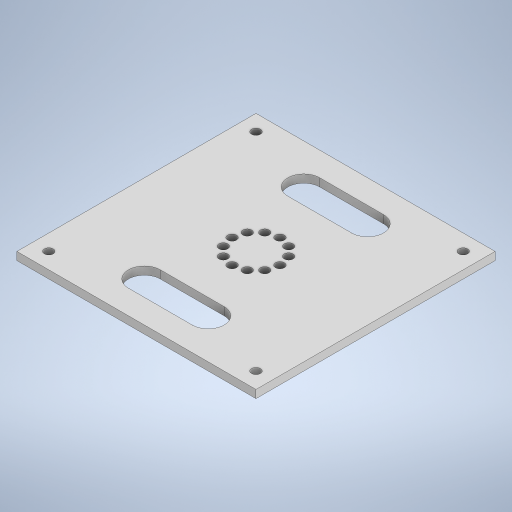
# Autodesk Inventor part: LowerBase
Saved by Autodesk Inventor 2023 (Build 270158000, 158)
## iProperties
Created: 2023-12-19
Part Number: LowerBase
Material: Generic
Document SubType Name: Modeling
Designer: Mustapha
Density: 1 g/cm^3
Appearance: Default
Author: Mustapha
Autodesk Inventor part; units mm, degrees
ref_plane "YZ Plane" through (0, 0, 0) normal (1, 0, 0) x (0, 1, 0)
ref_plane "XZ Plane" through (0, 0, 0) normal (0, 1, 0) x (-1, 0, 0)
ref_plane "XY Plane" through (0, 0, 0) normal (0, 0, 1) x (1, 0, 0)
sketch "Sketch1" plane through (0, 0, 0) normal (0, 1, 0) x (-1, 0, 0)
  line L0 (-75, 75) -> (75, 75)
  line L1 (75, 75) -> (75, -75)
  line L2 (75, -75) -> (-75, -75)
  line L3 (-75, -75) -> (-75, 75)
  line L4 (-75, 75) -> (75, -75) construction
  circle A0 centre (0, 0) radius 15
  circle A1 centre (15, 0) radius 2.75
  circle A2 centre (12.9904, 7.5) radius 2.75
  circle A3 centre (7.5, 12.9904) radius 2.75
  circle A4 centre (0, 15) radius 2.75
  circle A5 centre (-7.5, 12.9904) radius 2.75
  circle A6 centre (-12.9904, 7.5) radius 2.75
  line L5 (20, 50) -> (-20, 50) construction
  line L6 (20, 60) -> (-20, 60)
  line L7 (-20, 40) -> (20, 40)
  arc A7 (20, 40) -> (20, 60) centre (20, 50) ccw
  arc A8 (-20, 60) -> (-20, 40) centre (-20, 50) ccw
  line L8 (0, 0) -> (59.9777, 0)
  line L9 (20, -60) -> (-20, -60)
  line L10 (-20, -40) -> (20, -40)
  arc A9 (20, -60) -> (20, -40) centre (20, -50) ccw
  arc A10 (-20, -40) -> (-20, -60) centre (-20, -50) ccw
  circle A11 centre (65, 65) radius 2.75
  line L11 (0, 0) -> (0, -8.8495)
  circle A12 centre (65, -65) radius 2.75
  circle A13 centre (-65, 65) radius 2.75
  circle A14 centre (-65, -65) radius 2.75
  circle A15 centre (-15, 0) radius 2.75
  circle A16 centre (-12.9904, -7.5) radius 2.75
  circle A17 centre (-7.5, -12.9904) radius 2.75
  circle A18 centre (0, -15) radius 2.75
  circle A19 centre (7.5, -12.9904) radius 2.75
  circle A20 centre (12.9904, -7.5) radius 2.75
  point P0 (0, 50)
  point P1 (0, -50)
  point P2 (0, -4.4247)
  dimension "d2" = 30
  dimension "d0" = 150
  dimension "d1" = 150
  dimension "d3" = 5.5
  dimension "d6" = 360
  dimension "d10" = 40
  dimension "d11" = 20
  dimension "d12" = 40
  dimension "d13" = 5.5
  dimension "d14" = 10
  dimension "d15" = 10
  dimension "d16" = 20
  constraints: 26 end point, 20 centre point, 10 symmetric about line, 8 point on circle, 4 tangent, 3 horizontal, 3 midpoint, 3 parallel, 1 coincident, 1 horizontal alignment, 1 perpendicular, 1 vertical, 32 other
  measures "d0" distance between parallel lines of L3 L1
  measures "d1" distance of L0.end L1.end
  measures "d3" diameter of A1
  measures "d10" distance of L5.end L5.start
  measures "d11" distance between parallel lines of L7 L6
  measures "d12" distance between parallel lines of L8 L7
  measures "d13" diameter of A11
  measures "d14" distance from line of L1 A11.centre
  measures "d15" distance from line of L0 A11.centre
  measures "d16" horizontal distance of L6.end point (0, -4.425)
extrude "Extrusion1" add sketch "Sketch1" along normal blind 5 contours L0 L1 L2 L3 | A1 A0 A20 A19 A18 A17 A16 A15 A6 A5 A4 A3 A2
body "Solid1"
